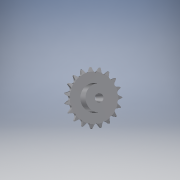
# Autodesk Inventor part: Sprocket
Saved by Autodesk Inventor 2018 (Build 220112000, 112)
## iProperties
Shininess: 64.0
Angle Display Precision: 2
Document Length Units: 11269
Document Angle Units: 11279
Document Time Units: 11290
Document Mass Units: 11283
Document Length Units Precision: 3
Document Angle Units Precision: 2
Compacted: True
Created: 2002-04-12
Part Number: Sprocket
Material: PAEK Plastic
Document SubType Name: Modeling
Designer: scotta
Density: 1.32 g/cm^3
Mass: 329.147 g
Surface Area: 147.659 cm^2
Volume: 41.8763 cm^3
Appearance: Smooth - White
Density: 0.0
Volumn: 0.0
Area: 0.0
PropertySet Name: Model Information
Control State: 0
Master: False
Checked Out: False
Author: scotta
Autodesk Inventor part; units mm, degrees
note: some values were not read from the file. Left out: dimensions or parameters whose unit could not be read.
ref_plane "YZ Plane" through (0, 0, 0) normal (1, 0, 0) x (0, 1, 0)
ref_plane "XZ Plane" through (0, 0, 0) normal (0, 1, 0) x (-1, 0, 0)
sketch "Sketch1" plane through (0, 0, 0) normal (0, 0, 1) x (1, 0, 0)
  circle A0 centre (0, 0) radius 17.5
  dimension "d0" = 35
  constraints: 1 centre point, 1 coincident
  measures "d0" diameter of A0
extrude "Extrusion1" add sketch "Sketch1" against normal blind 17
sketch "Sketch2" plane through (0, 0, 0) normal (0, 0, 1) x (1, 0, 0)
  circle A0 centre (0, 0) radius 41.8592
  circle A1 centre (0, 0) radius 31.75
  line L0 (0, 0) -> (0, 38.1088) construction
  arc A2 (-3.3822, 29.8361) -> (3.3822, 29.8361) centre (0, 31.75) ccw
  arc A3 (-5.2568, 33.1486) -> (-10.9601, 36.4744) centre (-10.9601, 29.9212) ccw
  line L1 (-3.3822, 29.8361) -> (-5.2568, 33.1486)
  line L2 (3.3822, 29.8361) -> (5.2568, 33.1486)
  line L3 (10.9601, 81.75) -> (-10.9601, 81.75)
  line L4 (-10.9601, 29.9212) -> (-10.9601, 29.7983)
  line L5 (-10.9601, 36.4744) -> (-10.9601, 81.75)
  line L6 (10.9601, 29.9212) -> (10.9601, 29.7983)
  line L7 (10.9601, 36.4744) -> (10.9601, 81.75)
  arc A4 (10.9601, 36.4744) -> (5.2568, 33.1486) centre (10.9601, 29.9212) ccw
  circle A5 centre (0, 0) radius 17.5 projected
  dimension "d3" = 83.7184
  dimension "d4" = 63.5
  dimension "d5" = 10.9601
  dimension "d6" = 10.9601
  dimension "d7" = 1.8288
  dimension "d8" = 1.8288
  dimension "d9" = 3.8862
  dimension "d10" = 6.5532
  dimension "d11" = 6.5532
  dimension "d12" = 50
  constraints: 16 end point, 9 point on circle, 6 parallel, 5 centre point, 4 tangent, 3 coincident, 2 collinear, 2 perpendicular, 1 concentric, 1 point on line, 1 vertical
  measures "d3" diameter of A0
  measures "d4" diameter of A1
  measures "d5" horizontal distance of point (10.96, 29.921) A1.start
  measures "d6" horizontal distance of point (-10.96, 29.921) A1.start
  measures "d7" vertical distance of point (10.96, 29.921) A1.start
  measures "d8" vertical distance of A1.start point (-10.96, 29.921)
  measures "d9" radius of A2
  measures "d10" radius of A4
  measures "d11" radius of A3
  measures "d12" distance from line of L3 A1.start
sketch "Sketch3" plane through (0, 0, 0) normal (1, 0, 0) x (0, 1, 0)
  line L0 (-35.5092, 0) -> (-46.8592, 0)
  line L1 (-46.8592, 0) -> (-46.8592, 7.2136)
  line L2 (-46.8592, 7.2136) -> (-35.5092, 7.2136)
  line L3 (-35.5092, 7.2136) -> (-41.8592, 6.023)
  line L4 (-41.8592, 6.023) -> (-41.8592, 1.1906)
  line L5 (-41.8592, 1.1906) -> (-35.5092, 0)
  line L6 (-17.5, 0) -> (17.5, 0) projected
  line L7 (0, 0) -> (0, 14.0847) construction
  line L8 (0, 0) -> (-72.931, 0)
  dimension "d13" = 1.1906
  dimension "d14" = 1.1906
  dimension "d15" = 6.35
  dimension "d16" = 5
  dimension "d17" = 7.2136
  dimension "d21" = 41.8592
  constraints: 16 end point, 3 parallel, 3 perpendicular, 1 collinear, 1 horizontal, 1 midpoint
  measures "d13" vertical distance of L2.end L3.end
  measures "d14" vertical distance of L4.end L0.start
  measures "d15" horizontal distance of L4.end L0.start
  measures "d16" distance from line of L1.end L4
  measures "d17" distance of L0.end L1.end
  measures "d21" distance between parallel lines of L7 L4
extrude "Sprocket Disc" add sketch "Sketch2" along normal blind 6 contours A0 L5 A3 L1 A1 L2 A4 L7 | L7 A4 L2 A1 L1 A3 L5 A0 | L2 A2 L1 A1 | A1 L1 A2 L2 | A5
chamfer "Sprocket Chamfer 1" distance 1.1906 distance2 6.35 1 edges at (-41.8592, 0, 6) measured on face at (14.0797, -39.4202, 4)
chamfer "Sprocket Chamfer 2" distance 6.35 distance2 1.1906 1 edges at (-41.8592, 0, 0) measured on face at (-16.3086, -29.3116, 0)
extrude "Tooth Cut" cut sketch "Sketch2" along normal blind 7.2136 contours L7 A4 L2 A1 L1 A3 L5 A0 | A0 L5 L3 L7 | L2 A2 L1 A1 picked at (-0.4791, 38.3699) picked at (-0.1516, 30.4418)
pattern_circular "Tooth Cut Array" count 19 over 360 about axis through (0, 0, 0) along (0, 0, 1) of "Tooth Cut"
sketch "Sketch4" plane through (0, 0, -17) normal (0, 0, -1) x (-1, 0, 0)
  circle A0 centre (0, 0) radius 17.5 projected
  circle A1 centre (0, 0) radius 6.35
  dimension "d32" = 12.7
  constraints: 1 centre point, 1 coincident
  measures "d32" diameter of A1
extrude "TaperBore" cut sketch "Sketch4" against normal through all draft -4 contours A1
sketch "Sketch5" plane through (0, 0, -17) normal (0, 0, -1) x (-1, 0, 0)
  circle A0 centre (0, 0) radius 17.5 projected
  circle A1 centre (0, 0) radius 22.225
  line L0 (0, 0) -> (0, 30.3364) construction
  line L1 (0, 0) -> (33.2732, -2.911) construction
  line L2 (0, 0) -> (-32.0919, -2.8077) construction
  point P0 (0, 22.225)
  point P1 (22.1404, -1.937)
  point P2 (-22.1404, -1.937)
  dimension "d35" = 95
  dimension "d36" = 95
  dimension "d37" = 44.45
  constraints: 6 end point, 3 point on circle, 3 point on line, 1 centre point, 1 coincident, 1 vertical
  measures "d35" angle of L1 L0
  measures "d36" angle of L2 L0
  measures "d37" diameter of A1
ref_plane "Work Plane3" through (0, 0, 3) normal (0, 0, 1) x (1, 0, 0)
equation "\"d3\" = OD"
equation "\"d5\" = Wx"
equation "\"d6\" = Wx"
equation "\"d7\" = Vy"
equation "\"d8\" = Vy"
equation "\"d9\" = R"
equation "\"d10\" = F"
equation "\"d11\" = F"
equation "\"d13\" = Chamfer_E"
equation "\"d14\" = Chamfer_E"
equation "\"d15\" = Chamfer_C"
equation "\"d17\" = T"
equation "\"d21\" = 0.5 * OD"
equation "\"d28\" = Chamfer_E"
equation "\"d29\" = Chamfer_C"
equation "\"d30\" = Chamfer_C"
equation "\"d31\" = Chamfer_E"
equation "\"d22\" = T"
equation "\"d37\" = HolePCD"
equation "\"Pitch_Dia\" = 77.1652"
equation "\"OD\" = 83.7184"
equation "\"T\" = 7.2136"
equation "\"R\" = 3.8862"
equation "\"Wx\" = 10.9601"
equation "\"Vy\" = 1.8288"
equation "\"Chamfer_C\" = 6.35"
equation "\"Chamfer_E\" = 1.19063"
equation "\"HubDepth\" = 25.4"
equation "\"HubDia\" = 63.5"
equation "\"TaperDia\" = 47.625"
equation "\"HoleDepth\" = 15.875"
equation "\"ThreadSize\" = 9.525"
equation "\"TappingDrillSize\" = 8.4328"
equation "\"HolePCD\" = 44.45"
body "Solid1"
